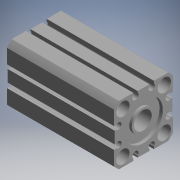
# Autodesk Inventor part: CDQSB25-40DM(1_0)_BODY
Saved by Autodesk Inventor 2017.3 (Build 213256000, 256)
## iProperties
Part Number: CDQSB25-40DM(1_0)_BODY
Material: Generic
Catalog Web Link: www.cadenas.de
Description: CQS/CDQS BODY-Compact Cylinder:Standard Type Double Acting,Single Rod
Vendor: SMC
Document SubType Name: Modeling
Designer: partserver
Manufacturer: SMC
Mass: 69.8434 g
Surface Area: 298.631 cm^2
Volume: 69.8434 cm^3
Density: 1 g/cm^3
Appearance: PSOLRGB-192-192-192
Category: PARTsolutions
Company: SMC
Title: CDQSB25-40DM_BODY
Author: Cadenas PARTsolutions
Comments: Compact Cylinder:Standard Type Double Acting,Single Rod
PSOL_IDENT_0: {$CADENAS_DATA\23d-libs\smc_jp\actuator\compact_cylinder\cqs\cqs\parts\cqs_body.prj},286 {VTYP=3D},{
PSOL_IDENT_1: NB=CDQSB25-40DM(1_0)_BODY},{LINA=CDQSB25-40DM_BODY},{NN=CQS/CDQS BODY},{DATE=29.10.2021 06:14:23},{G
PSOL_IDENT_2: EOMDATE=29.10.2019 09:23:28},{VERSION=},{LINEID=40},{WBVAR=TYPE,MOUNT,MAGNET,STROKE,STOP,BODY,AUTOSW
PSOL_IDENT_3: ITCH,OMSC1,OMSC2,OMSC3,OMSC4,OMSC5,OMSC6,OMSC7,THREAD},{WBNUMERIC=STROKE}  {NB=CDQSB25-40DM(1_0)_BOD
PSOL_IDENT_4: Y},{LINA=CDQSB25-40DM_BODY},{KT=DUMMY},{BORE=25},{TYPE=},{TP=A},{MOUNT=B},{MAGNET=D},{STROKE=40},{ST
PSOL_IDENT_5: ROKEX2=40},{STOP=1},{ACTION=(D) Double acting},{BODY=M},{BODYX='','(-) Standard (Rod end female thre
PSOL_IDENT_6: ad)','C','(C) With rubber bumper','M','(M) Rod end male thread','F','(F) Boss on head side','CM','(C
PSOL_IDENT_7: M) With rubber bumper & Rod end male thread','FC','(FC) Boss on head side & With rubber bumper','FM'
PSOL_IDENT_8: ,'(FM) Boss on head side & Rod end male thread','FCM','(FCM) Boss on head side & With rubber bumper
PSOL_IDENT_9: & Rod end male thread'},{ORDER=CDQSB25-40DM},{AUTOSWITCH=},{AUTOSWITCHX='','(-) Without autoswitch','
PSOL_IDENT_10: -M9NV','M9NV','-M9PV','M9PV','-M9BV','M9BV','-M9N','M9N','-M9P','M9P','-M9B','M9B','-M9NWV','M9NWV','
PSOL_IDENT_11: -M9PWV','M9PWV','-M9BWV','M9BWV','-M9NW','M9NW','-M9PW','M9PW','-M9BW','M9BW','-M9NAV','M9NAV','-M9P
PSOL_IDENT_12: AV','M9PAV','-M9BAV','M9BAV','-M9NA','M9NA','-M9PA','M9PA','-M9BA','M9BA','-A96V','A96V','-A93V','A9
PSOL_IDENT_13: 3V','-A90V','A90V','-A96','A96','-A93','A93','-A90','A90','-P3DWA','P3DWA','-P3DWASC','P3DWASC','-P3
PSOL_IDENT_14: DWASE','P3DWASE'},{OMSC1=},{OMSC1X= '','N/A' },{OMSC2=},{OMSC2X='','(-) Without order','-XB9','(-XB9
PSOL_IDENT_15: ) Low speed cylinder (10 to 50 mm/s)','-XB13','(-XB13) Low speed cylinder (5 to 50 mm/s)'},{OMSC3=},
PSOL_IDENT_16: {OMSC3X='','(-) Without order','-XC6','(-XC6) Piston rod, retaining ring, rod end nut made of stainl
PSOL_IDENT_17: ess steel','-X271','(-X271) Fluororubber seals'},{OMSC4=},{OMSC4X='','(-) Without order','-XC36','(-
PSOL_IDENT_18: XC36) With boss in rod side'},{OMSC5=},{OMSC5X='','(-) Without order','-XC85','(-XC85) Grease for fo
PSOL_IDENT_19: od processing equipment'},{OMSC6=},{OMSC6X='','(-) Without order','-X1876','(-X1876) With concave sh
PSOL_IDENT_20: ape end boss on the cylinder tube head side'},{OMSC7=},{OMSC7X='','N/A'},{THREAD=0},{A=37.5},{AA1=27
PSOL_IDENT_21: .5},{AA2=37.5},{AA3=59.0},{B=32.5},{BB1=22.5},{BB2=32.5},{BB3=44.0},{F=5.5},{FF1=5.5},{FF2=5.5},{FF3=
PSOL_IDENT_22: 9.0},{D=12},{E=40},{I=52},{K=10},{M=28.0},{N=5.4},{OA=M6x1.0},{OARA=6},{OARP=1.0},{OB=9.0},{TH=15},{
PSOL_IDENT_23: Q=9.0},{RA=10},{RB=7},{L1=11},{L2=8.0},{AD=11.0},{AD1=7.0},{AD2=11.0},{AD3=10.0},{AD4=14.0},{BD=9.5}
PSOL_IDENT_24: ,{BD1=5.5},{BD2=9.5},{BD3=14.0},{BD4=18.0},{G=2.0},{XC36TH9=15},{XC36G=2.0},{X187610=23.8},{X1876G=1
PSOL_IDENT_25: .4},{SLIPA=0.500},{SLIPB=2.150},{SLIPE=15.000},{SLIPF=26.000}
NB: CDQSB25-40DM(1_0)_BODY
NN: CQS/CDQS BODY
NT: Compact Cylinder:Standard Type Double Acting,Single Rod
NBSYN: $ORDER.($STOP._$THREAD.)_BODY
LINA: CDQSB25-40DM_BODY
CATALOG: SMC (JP
BORE: 25
TYPE: (-) None
MOUNT: (B) Through-hole/Both ends tapped common (Standard)
MAGNET: (D) With magnet
STROKE: 40
STOP: Manufacturable stroke
ACTION: (D) Double acting
BODY: (M) Rod end male thread
AUTOSWITCH: (-) Without autoswitch
OMSC1: N/A
OMSC2: (-) Without order
OMSC3: (-) Without order
OMSC4: (-) Without order
OMSC5: (-) Without order
OMSC6: (-) Without order
OMSC7: N/A
THREAD: on
A: 37.5
B: 32.5
F: 5.5
D: 12
E: 40
I: 52
K: 10
M: 28
N: 5.4
OA: M6x1.0
OB: 9
TH: 15
Q: 9
RA: 10
RB: 7
L1: 11
L2: 8
AD1: 7
AD2: 11
AD3: 10
AD4: 14
BD1: 5.5
BD2: 9.5
BD3: 14
BD4: 18
G: 2
XC36TH9: 15
XC36G: 2
X187610: 23.8
X1876G: 1.4
SLIPA: 0.5
SLIPB: 2.15
SLIPE: 15
SLIPF: 26
SUPPLIER: SMC
ARTICLENO: CDQSB25-40DM(1_0)_BODY
BOMINFO: CDQSB25-40DM_BODY
CREATOR: CADENAS GmbH
Autodesk Inventor part; units mm, degrees
sketch "Sketch_13" plane through (0, 0, 0) normal (1, 0, 0) x (0, 1, 0)
  line L0 (16.6132, 20) -> (7, 20)
  line L1 (7, 20) -> (7, 18.4697)
  arc A0 (4, 18.4697) -> (7, 18.4697) centre (5.5, 17) ccw
  line L2 (4, 18.4697) -> (4, 19.5)
  line L3 (4, 19.5) -> (-4, 19.5)
  line L4 (-4, 19.5) -> (-4, 18.4697)
  arc A1 (-7, 18.4697) -> (-4, 18.4697) centre (-5.5, 17) ccw
  line L5 (-7, 18.4697) -> (-7, 20)
  line L6 (-7, 20) -> (-16.6132, 20)
  arc A2 (-16.6132, 20) -> (-20, 16.6132) centre (0, 0) ccw
  line L7 (-20, 16.6132) -> (-20, 7)
  line L8 (-20, 7) -> (-18.4697, 7)
  arc A3 (-18.4697, 4) -> (-18.4697, 7) centre (-17, 5.5) ccw
  line L9 (-18.4697, 4) -> (-19.5, 4)
  line L10 (-19.5, 4) -> (-19.5, -4)
  line L11 (-19.5, -4) -> (-18.4697, -4)
  arc A4 (-18.4697, -7) -> (-18.4697, -4) centre (-17, -5.5) ccw
  line L12 (-18.4697, -7) -> (-20, -7)
  line L13 (-20, -7) -> (-20, -16.6132)
  arc A5 (-20, -16.6132) -> (-16.6132, -20) centre (0, 0) ccw
  line L14 (-16.6132, -20) -> (-7, -20)
  line L15 (-7, -20) -> (-7, -18.4697)
  arc A6 (-4, -18.4697) -> (-7, -18.4697) centre (-5.5, -17) ccw
  line L16 (-4, -18.4697) -> (-4, -19.5)
  line L17 (-4, -19.5) -> (4, -19.5)
  line L18 (4, -19.5) -> (4, -18.4697)
  arc A7 (7, -18.4697) -> (4, -18.4697) centre (5.5, -17) ccw
  line L19 (7, -18.4697) -> (7, -20)
  line L20 (7, -20) -> (16.6132, -20)
  arc A8 (16.6132, -20) -> (20, -16.6132) centre (0, 0) ccw
  line L21 (20, -16.6132) -> (20, -7)
  line L22 (20, -7) -> (18.4697, -7)
  arc A9 (18.4697, -4) -> (18.4697, -7) centre (17, -5.5) ccw
  line L23 (18.4697, -4) -> (19.5, -4)
  line L24 (19.5, -4) -> (19.5, 4)
  line L25 (19.5, 4) -> (18.4697, 4)
  arc A10 (18.4697, 7) -> (18.4697, 4) centre (17, 5.5) ccw
  line L26 (18.4697, 7) -> (20, 7)
  line L27 (20, 7) -> (20, 16.6132)
  arc A11 (20, 16.6132) -> (16.6132, 20) centre (0, 0) ccw
  constraints: 56 end point, 24 point on circle, 12 centre point
extrude "Extrusion1" add sketch "Sketch_13" along normal blind 72.5
sketch "Sketch_2" plane through (0, 0, 14) normal (0, 0, 1) x (1, 0, 0)
  line L0 (72.5, 14) -> (0, 14)
  line L1 (0, 14) -> (0, 18.5)
  line L2 (0, 18.5) -> (7, 18.5)
  line L3 (7, 18.5) -> (7, 17)
  line L4 (7, 17) -> (7.5415, 16.4585)
  line L5 (7.5415, 16.4585) -> (17, 16.4585)
  line L6 (17, 16.4585) -> (17.1394, 16.7)
  line L7 (17.1394, 16.7) -> (55.3606, 16.7)
  line L8 (55.3606, 16.7) -> (55.5, 16.4585)
  line L9 (55.5, 16.4585) -> (64.9585, 16.4585)
  line L10 (64.9585, 16.4585) -> (65.5, 17)
  line L11 (65.5, 17) -> (65.5, 18.5)
  line L12 (65.5, 18.5) -> (72.5, 18.5)
  line L13 (72.5, 18.5) -> (72.5, 14)
  line L14 (72.5, 14) -> (0, 14)
  constraints: 30 end point
revolve "Revolution1" cut sketch "Sketch_2" angle 360 about axis through (72.5, 14, 14) along (1, 0, 0)
thread "Thread1" size "M6x1" class "6H" standard "ISO Metric profile" full length
thread "Thread2" size "M6x1" class "6H" standard "ISO Metric profile" full length
pattern_linear "Rectangular Pattern1" count 2 spacing 28 along (0, 0, -1) count 2 spacing 28 along (0, -1, 0) of "Revolution1"
sketch "Sketch_5" plane through (0, 0, 0) normal (0, 0, 1) x (1, 0, 0)
  line L0 (61.25, 0) -> (-2, 0)
  line L1 (-2, 0) -> (-2, 6)
  line L2 (-2, 6) -> (16.25, 6)
  line L3 (16.25, 6) -> (16.25, 12.5)
  line L4 (16.25, 12.5) -> (61.25, 12.5)
  line L5 (61.25, 12.5) -> (61.25, 0)
  line L6 (61.25, 0) -> (-2, 0)
  constraints: 14 end point
revolve "Revolution2" cut sketch "Sketch_5" angle 360 about axis through (61.25, 0, 0) along (1, 0, 0)
sketch "Sketch_4" plane through (0, 0, 0) normal (0, 0, 1) x (1, 0, 0)
  line L0 (9, 13.3066) -> (9, 19.5)
  line L1 (9, 19.5) -> (11.5, 19.5)
  line L2 (11.5, 19.5) -> (11.067, 19.067)
  line L3 (11.067, 19.067) -> (11.067, 14.5)
  line L4 (11.067, 14.5) -> (9, 13.3066)
  line L5 (9, 13.3066) -> (9, 19.5)
  constraints: 12 end point
revolve "Revolution3" cut sketch "Sketch_4" angle 360 about axis through (9, 13.3066, 0) along (0, -1, 0)
thread "Thread3" size "M5x0.8" class "6H" standard "ISO Metric profile" full length
sketch "Sketch_6" plane through (0, 0, 0) normal (0, 0, 1) x (1, 0, 0)
  line L0 (67, 13.3066) -> (67, 19.5)
  line L1 (67, 19.5) -> (69.5, 19.5)
  line L2 (69.5, 19.5) -> (69.067, 19.067)
  line L3 (69.067, 19.067) -> (69.067, 14.5)
  line L4 (69.067, 14.5) -> (67, 13.3066)
  line L5 (67, 13.3066) -> (67, 19.5)
  constraints: 12 end point
revolve "Revolution4" cut sketch "Sketch_6" angle 360 about axis through (67, 13.3066, 0) along (0, -1, 0)
thread "Thread4" size "M5x0.8" class "6H" standard "ISO Metric profile" full length
sketch "Sketch_26" plane through (0, 0, 0) normal (1, 0, 0) x (0, 1, 0)
  circle A0 centre (0, 0) radius 13
  circle A1 centre (0, 0) radius 7.5
  constraints: 2 centre point
extrude "Extrusion2" cut sketch "Sketch_26" along normal blind 2.15
sketch "Sketch_27" plane through (0, 0, 0) normal (1, 0, 0) x (0, 1, 0)
  circle A0 centre (0, 0) radius 7.5
  constraints: 1 centre point
extrude "Extrusion3" cut sketch "Sketch_27" along normal blind 0.5
ref_plane "BODY_DUMMY_XY" through (0, 0, 0) normal (-1, 0, 0) x (0, 0, -1)
ref_plane "BODY_DUMMY_YZ" through (0, 0, 0) normal (0, 0, -1) x (0, -1, 0)
ref_plane "BODY_DUMMY_ZX" through (0, 0, 0) normal (0, -1, 0) x (-1, 0, 0)
ref_plane "BODY_MOUBT1_XY" through (0, 0, 0) normal (-1, 0, 0) x (0, 0, -1)
ref_plane "BODY_MOUBT1_YZ" through (0, 0, 0) normal (0, 0, -1) x (0, -1, 0)
ref_plane "BODY_MOUBT1_ZX" through (0, 0, 0) normal (0, -1, 0) x (-1, 0, 0)
ref_plane "BODY_MOUBT2_XY" through (72.5, 0, 0) normal (1, 0, 0) x (0, 0, -1)
ref_plane "BODY_MOUBT2_YZ" through (72.5, 0, 0) normal (0, 0, -1) x (0, 1, 0)
ref_plane "BODY_MOUBT2_ZX" through (72.5, 0, 0) normal (0, 1, 0) x (1, 0, 0)
ref_plane "BODY_ROD_XY" through (0, 0, 0) normal (-1, 0, 0) x (0, 0, -1)
ref_plane "BODY_ROD_YZ" through (0, 0, 0) normal (0, 0, -1) x (0, -1, 0)
ref_plane "BODY_ROD_ZX" through (0, 0, 0) normal (0, -1, 0) x (-1, 0, 0)
ref_plane "BODY_SWA_XY" through (11, -5.5, 17) normal (-1, 0, 0) x (0, 0, -1)
ref_plane "BODY_SWA_YZ" through (11, -5.5, 17) normal (0, 0, -1) x (0, -1, 0)
ref_plane "BODY_SWA_ZX" through (11, -5.5, 17) normal (0, -1, 0) x (-1, 0, 0)
ref_plane "BODY_SWB_XY" through (63, 5.5, 17) normal (1, 0, 0) x (0, 0, -1)
ref_plane "BODY_SWB_YZ" through (63, 5.5, 17) normal (0, 0, -1) x (0, 1, 0)
ref_plane "BODY_SWB_ZX" through (63, 5.5, 17) normal (0, 1, 0) x (1, 0, 0)
body "Solid1"
